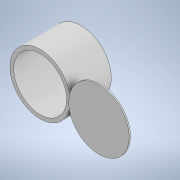
# Autodesk Inventor part: box
Saved by Autodesk Inventor 2021 (Build 250183000, 183)
## iProperties
Created: 2023-05-14
Part Number: box
Material: Generic
Document SubType Name: Modeling
Designer: Sahil Nadaf
Density: 1 g/cm^3
Appearance: Default
Author: Sahil Nadaf
Autodesk Inventor part; units mm, degrees
ref_plane "YZ Plane" through (0, 0, 0) normal (1, 0, 0) x (0, 1, 0)
ref_plane "XZ Plane" through (0, 0, 0) normal (0, 1, 0) x (-1, 0, 0)
ref_plane "XY Plane" through (0, 0, 0) normal (0, 0, 1) x (1, 0, 0)
sketch "Sketch1" plane through (0, 0, 0) normal (0, 0, 1) x (1, 0, 0)
  circle A0 centre (0, 0) radius 228.6
  dimension "d0" = 457.2
  constraints: 1 centre point, 1 coincident
  measures "d0" diameter of A0
extrude "Extrusion1" add sketch "Sketch1" along normal blind 304.8
sketch "Sketch2" plane through (0, 0, 304.8) normal (0, 0, 1) x (1, 0, 0)
  point P0 (0, 0)
hole "Hole1" at (0, 0, 304.8) direction (0, 0, 1) diameter 457.2 end through all
sketch "Sketch3" plane through (0, 0, 0) normal (0, 0, -1) x (-1, 0, 0)
  circle A0 centre (0, 0) radius 228.6
  dimension "d10" = 457.2
  constraints: 1 centre point, 1 coincident
  measures "d10" diameter of A0
hole "Hole2" at (0, 0, 0) direction (0, 0, -1) diameter 457.2 end through all
sketch "Sketch4" plane through (0, 0, 304.8) normal (0, 0, 1) x (1, 0, 0)
  circle A0 centre (0, 0) radius 200
  dimension "d18" = 400
  constraints: 1 centre point, 1 coincident
  measures "d18" diameter of A0
hole "Hole3" at (0, 0, 304.8) direction (0, 0, -1) diameter 400 end through all
sketch "Sketch5" plane through (0, 0, 0) normal (0, 0, -1) x (-1, 0, 0)
  circle A0 centre (0, 0) radius 228.6
  dimension "d26" = 457.2
  constraints: 1 centre point, 1 coincident
  measures "d26" diameter of A0
extrude "Extrusion2" add sketch "Sketch5" along normal blind 5
sketch "Sketch6" plane through (0, 0, 304.8) normal (0, 0, 1) x (1, 0, 0)
  circle A0 centre (0, 0) radius 228.6 projected
  line L0 (228.6, 0) -> (455.2, 0)
  circle A1 centre (455.2, 0) radius 228.6
  point P0 (227.6, -21.3588)
  point P1 (227.6, 21.3588)
  dimension "d29" = 226.6
  dimension "d30" = 457.2
  constraints: 2 end point, 1 centre point, 1 coincident, 1 horizontal, 2 other
  measures "d29" distance of L0.start L0.end
  measures "d30" diameter of A1
extrude "Extrusion3" add sketch "Sketch6" along normal blind 10 contours A0 A1 picked at (531.7419, 7.0282)
body "Solid1"
